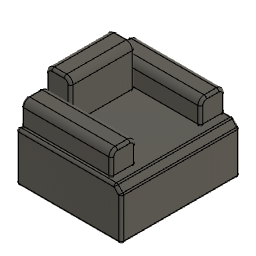
rgiro_yamazen_sofa_single (Autodesk Fusion 360 design; units mm, degrees)
Autodesk Fusion 360 part; units mm, degrees
sketch "Sketch1" plane through (0, 0, 0) normal (0, 0, 1) x (1, 0, 0)
  line L0 (425, -480) -> (-425, -480)
  line L1 (-425, -480) -> (-425, 480)
  line L2 (-425, 480) -> (425, 480)
  line L3 (425, 480) -> (425, -480)
  line L4 (425, -480) -> (-425, 480) construction
  line L5 (-425, -480) -> (425, 480) construction
  line L6 (-405, -460) -> (325, -460)
  line L7 (325, -460) -> (325, -260)
  line L8 (325, -260) -> (-405, -260)
  line L9 (-405, -260) -> (-405, -460)
  line L10 (-405, -260) -> (-205, -260)
  line L11 (-205, -260) -> (-205, 260)
  line L12 (-205, 260) -> (-405, 260)
  line L13 (-405, 260) -> (-405, -260)
  line L14 (-405, 260) -> (325, 260)
  line L15 (325, 260) -> (325, 460)
  line L16 (325, 460) -> (-405, 460)
  line L17 (-405, 460) -> (-405, 260)
  dimension "d1" = 960
  dimension "d2" = 850
  dimension "d3" = 20
  dimension "d4" = 20
  dimension "d5" = 20
  dimension "d6" = 200
  dimension "d7" = 200
  dimension "d8" = 100
  constraint perpendicular L0 L1
  constraint parallel L0 L2
  constraint parallel L1 L3
  constraint horizontal L0
  constraint coincident L4 origin
  constraint coincident L5 origin
  constraint horizontal L6
  constraint vertical L7
  constraint horizontal L8
  constraint vertical L9
  constraint horizontal L10
  constraint vertical L11
  constraint horizontal L12
  constraint vertical L13
  constraint horizontal L14
  constraint vertical L15
  constraint horizontal L16
  constraint vertical L17
  constraint collinear L9 L13
  constraint collinear L9 L17
  constraint collinear L7 L15
  constraint equal L7 L15
  constraint collinear L8 L10
  constraint collinear L12 L14
  measures "d1" distance of L0.start L2.end
  measures "d2" distance of L0.start L0.end
  measures "d3" distance of L1 L6.start
  measures "d4" distance of L0 L6
  measures "d5" distance of L2 L16
  measures "d6" distance of L6.end L7.end
  measures "d7" distance of L8.end L10.end
  measures "d8" distance of L3 L7
extrude "Extrude1" add sketch "Sketch1" along normal blind 400 contours L0 L1 L2 L3 | L6 L7 L8 L9 L10 | L8 L10 L11 L12 L13 L14 | L12 L14 L15 L16 L17 makes body 1
sketch "Sketch2" plane through (0, 0, 400) normal (0, 0, 1) x (-1, 0, 0)
  line L0 (-425, -480) -> (425, -480)
  line L1 (425, -480) -> (425, 480)
  line L2 (425, 480) -> (-425, 480)
  line L3 (-425, 480) -> (-425, -480)
  line L4 (405, 460) -> (-325, 460)
  line L5 (-325, 260) -> (405, 260)
  line L6 (405, 260) -> (405, 460)
  line L7 (-325, 460) -> (-325, 260)
  line L8 (405, -460) -> (405, -260)
  line L9 (405, -260) -> (-325, -260)
  line L10 (-325, -460) -> (405, -460)
  line L11 (-325, -260) -> (-325, -460)
extrude "Extrude2" add sketch "Sketch2" along normal blind 200 separate body contours L4 L5 L6 L7 | L8 L9 L10 L11 makes body 2 at (81.6667, -393.3333, 400) makes body 3 at (-161.6667, 393.3333, 400)
sketch "Sketch3" plane through (0, 0, 400) normal (0, 0, 1) x (-1, 0, 0)
  line L0 (-425, -480) -> (425, -480)
  line L1 (425, -480) -> (425, 480)
  line L2 (425, 480) -> (-425, 480)
  line L3 (-425, 480) -> (-425, -480)
  line L4 (205, 260) -> (205, -260)
  line L5 (205, -260) -> (405, -260)
  line L6 (405, 260) -> (205, 260)
  line L7 (405, -260) -> (405, 260)
extrude "Extrude3" add sketch "Sketch3" along normal blind 340 separate body contours L4 L5 L6 L7 makes body 4
chamfer "Chamfer2" distance 50 angle 45 1 edges at (425, 0, 400) on bodies 1
fillet "Fillet2" radius 20 7 faces at (425, 160, 116.6667) (391.6667, 160, 383.3333) (125, 480, 133.3333) (-425, -160, 133.3333) (125, -480, 133.3333) (-141.6667, -160, 0) (-158.3333, 160, 400) on bodies 1
fillet "Fillet3" radius 50 6 edges at (-40, -460, 600) (-40, -260, 600) (-40, 260, 600) (-40, 460, 600) (-205, 0, 740) (-405, 0, 740) on bodies 2 3 4
fillet "Fillet4" radius 20 21 faces at (-405, -326.6667, 450) (-161.6667, -460, 450) (-161.6667, -419.4626, 599.0964) (81.6667, -376.6667, 600) (81.6667, -300.5374, 599.0964) (81.6667, -260, 450) (325, -393.3333, 450) (-161.6667, 260, 450) (-161.6667, 300.5374, 599.0964) (-161.6667, 376.6667, 600) (81.6667, 432.9113, 594.4418) (-161.6667, 460, 500) (325, 326.6667, 450) (-405, 393.3333, 450) (-205, -86.6667, 593.3333) (-218.8133, -86.6667, 724.504) (-288.3333, -86.6667, 740) (-377.9113, 86.6667, 734.4418) (-405, 86.6667, 593.3333) (-271.6667, 260, 496.6667) (-338.3333, -260, 593.3333) on bodies 2 3 4
